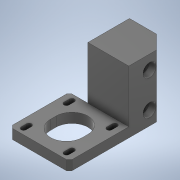
# Autodesk Inventor part: ymotorholder
Saved by Autodesk Inventor 2020.2 (Build 242310000, 310)
## iProperties
Created: 2020-08-06
Part Number: ymotorholder
Material: Generic
Document SubType Name: Modeling
Designer: JK
Density: 1 g/cm^3
Appearance: Smooth - Black
Author: JK
Autodesk Inventor part; units mm, degrees
ref_plane "YZ Plane" through (0, 0, 0) normal (1, 0, 0) x (0, 1, 0)
ref_plane "XZ Plane" through (0, 0, 0) normal (0, 1, 0) x (-1, 0, 0)
ref_plane "XY Plane" through (0, 0, 0) normal (0, 0, 1) x (1, 0, 0)
sketch "Sketch1" plane through (0, 0, 0) normal (0, 1, 0) x (-1, 0, 0)
  line L0 (-21.5, 21.5) -> (21.5, 21.5)
  line L1 (21.5, 21.5) -> (21.5, -21.5)
  line L2 (21.5, -21.5) -> (-21.5, -21.5)
  line L3 (-21.5, -21.5) -> (-21.5, 21.5)
  line L4 (-21.5, 21.5) -> (21.5, -21.5) construction
  line L5 (21.5, 21.5) -> (-21.5, -21.5) construction
  circle A0 centre (0, 0) radius 11.5
  circle A1 centre (15.5, 15.5) radius 1.8
  circle A2 centre (-15.5, 15.5) radius 1.8
  circle A3 centre (-15.5, -15.5) radius 1.8
  circle A4 centre (15.5, -15.5) radius 1.8
  dimension "d0" = 23
  dimension "d1" = 43
  dimension "d2" = 43
  dimension "d3" = 3.6
  dimension "d5" = 31
  dimension "d6" = 31
  constraints: 12 end point, 5 centre point, 4 point on line, 3 equal radius, 2 midpoint, 2 parallel, 2 vertical alignment, 1 coincident, 1 horizontal, 1 perpendicular
  measures "d0" diameter of A0
  measures "d1" distance of L1.end L2.end
  measures "d2" distance of L0.end L1.end
  measures "d3" diameter of A1
  measures "d5" distance of A4.centre A1.centre
  measures "d6" distance of A3.centre A4.centre
extrude "Extrusion1" add sketch "Sketch1" along normal blind 7
sketch "Sketch6" plane through (0, 0, 0) normal (0, -1, 0) x (1, 0, 0)
  line L0 (21.5, -21.5) -> (-21.5, -21.5) projected
  line L1 (-8, -21.5) -> (-8, -51.5)
  line L2 (21.5, -21.5) -> (-8, -21.5)
  line L3 (-8, -21.5) -> (-8, -51.5)
  line L4 (-8, -51.5) -> (21.5, -51.5)
  line L5 (21.5, -51.5) -> (21.5, -21.5)
  point P0 (0, 0)
  dimension "d26" = 8
  dimension "d27" = 30
  constraints: 10 end point, 2 parallel, 1 horizontal, 1 perpendicular, 1 point on line, 1 vertical
  measures "d26" distance from line of point (0, 0) L1
  measures "d27" distance of L1.start L1.end
extrude "Extrusion5" add sketch "Sketch6" against normal blind 45
chamfer "Chamfer1" distance 2 angle 45 3 edges at (21.5, 3.5, 21.5) (-21.5, 3.5, 21.5) (-21.5, 3.5, -21.5)
sketch "Sketch7" plane through (21.5, 0, -51.5) normal (1, 0, 0) x (0, 0, -1)
  circle A0 centre (-15, 35) radius 2.8
  circle A1 centre (-15, 10) radius 2.8
  line L0 (0, 0) -> (0, 45) projected
  line L1 (-71, 7) -> (-30, 7) projected
  line L2 (-71, 0) -> (0, 0) projected
  line L3 (-30, 45) -> (0, 45) projected
  point P0 (-51.5, 0)
  dimension "d33" = 5.6
  dimension "d34" = 5.6
  dimension "d35" = 15
  dimension "d37" = 10
  dimension "d38" = 10
  constraints: 2 centre point
  measures "d33" diameter of A0
  measures "d34" diameter of A1
  measures "d35" distance from line of L0 A0.centre
  measures "d37" distance from line of L2 A1.centre
  measures "d38" distance from line of L3 A0.centre
extrude "Extrusion6" cut sketch "Sketch7" against normal through all
sketch "Sketch8" plane through (21.5, 0, -51.5) normal (1, 0, 0) x (0, 0, -1)
  circle A0 centre (-15, 35) radius 2.8 projected
  circle A1 centre (-15, 35) radius 4.75
  circle A2 centre (-15, 10) radius 2.8 projected
  circle A3 centre (-15, 10) radius 4.75
  point P0 (-51.5, 0)
  dimension "d41" = 9.5
  dimension "d42" = 9.5
  constraints: 2 centre point, 2 coincident
  measures "d41" diameter of A1
  measures "d42" diameter of A3
extrude "Extrusion7" cut sketch "Sketch8" against normal blind 5 contours A0 | A1 | A2 | A3
chamfer "Chamfer2" distance 10 angle 45 1 edges at (21.5, 22.5, -51.5)
sketch "Sketch9" plane through (0, 0, 0) normal (0, -1, 0) x (1, 0, 0)
  line L0 (13.7, 17.5) -> (17.3, 17.5)
  line L1 (17.3, 17.5) -> (17.3, 13.5)
  line L2 (17.3, 13.5) -> (13.7, 13.5)
  line L3 (13.7, 13.5) -> (13.7, 17.5)
  circle A0 centre (15.5, 15.5) radius 1.8 projected
  line L4 (13.7, 17.5) -> (17.3, 13.5) construction
  line L5 (17.3, 17.5) -> (13.7, 13.5) construction
  line L6 (13.7, -13.5) -> (17.3, -13.5)
  line L7 (17.3, -13.5) -> (17.3, -17.5)
  line L8 (17.3, -17.5) -> (13.7, -17.5)
  line L9 (13.7, -17.5) -> (13.7, -13.5)
  circle A1 centre (15.5, -15.5) radius 1.8 projected
  line L10 (13.7, -13.5) -> (17.3, -17.5) construction
  line L11 (17.3, -13.5) -> (13.7, -17.5) construction
  line L12 (-17.3, 17.5) -> (-13.7, 17.5)
  line L13 (-13.7, 17.5) -> (-13.7, 13.5)
  line L14 (-13.7, 13.5) -> (-17.3, 13.5)
  line L15 (-17.3, 13.5) -> (-17.3, 17.5)
  circle A2 centre (-15.5, 15.5) radius 1.8 projected
  line L16 (-17.3, 17.5) -> (-13.7, 13.5) construction
  line L17 (-13.7, 17.5) -> (-17.3, 13.5) construction
  line L18 (-17.3, -13.5) -> (-13.7, -13.5)
  line L19 (-13.7, -13.5) -> (-13.7, -17.5)
  line L20 (-13.7, -17.5) -> (-17.3, -17.5)
  line L21 (-17.3, -17.5) -> (-17.3, -13.5)
  circle A3 centre (-15.5, -15.5) radius 1.8 projected
  line L22 (-17.3, -13.5) -> (-13.7, -17.5) construction
  line L23 (-13.7, -13.5) -> (-17.3, -17.5) construction
  circle A4 centre (15.5, 17.5) radius 1.8
  circle A5 centre (15.5, -17.5) radius 1.8
  circle A6 centre (15.5, -13.5) radius 1.8
  circle A7 centre (-15.5, -17.5) radius 1.8
  circle A8 centre (-15.5, -13.5) radius 1.8
  circle A9 centre (-15.5, 13.5) radius 1.8
  circle A10 centre (-15.5, 17.5) radius 1.8
  circle A11 centre (15.5, 13.5) radius 1.8
  point P0 (0, 0)
  point P1 (-17.3, 17.5)
  point P2 (13.7, 17.5)
  point P3 (17.3, 13.5)
  dimension "d48" = 4
  dimension "d49" = 4
  constraints: 48 end point, 16 midpoint, 8 parallel, 4 horizontal, 4 perpendicular, 3 point on line, 3 tangent, 2 horizontal alignment, 1 centre point, 21 other
  measures "d48" distance of L2.end L0.start
  measures "d49" distance of L6.end L7.end
extrude "Extrusion8" cut sketch "Sketch9" against normal blind 10
sketch "Sketch10" plane through (0, 0, 0) normal (0, -1, 0) x (1, 0, 0)
  line L0 (-11.5, 2) -> (11.5, 2)
  line L1 (11.5, 2) -> (11.5, -2)
  line L2 (11.5, -2) -> (-11.5, -2)
  line L3 (-11.5, -2) -> (-11.5, 2)
  line L4 (-11.5, 2) -> (11.5, -2) construction
  line L5 (11.5, 2) -> (-11.5, -2) construction
  circle A0 centre (0, -2) radius 11.5
  circle A1 centre (0, 2) radius 11.5
  circle A2 centre (0, 0) radius 11.5 projected
  point P0 (11.3248, 2)
  point P1 (-11.3248, 2)
  point P2 (-11.3248, -2)
  point P3 (11.3248, -2)
  point P4 (-11.5, 0)
  point P5 (11.5, 0)
  dimension "d52" = 4
  constraints: 12 end point, 4 midpoint, 2 parallel, 1 horizontal, 1 perpendicular, 1 tangent, 6 other
  measures "d52" distance of point (0, -2) point (0, 2)
extrude "Extrusion9" cut sketch "Sketch10" against normal blind 10
sketch "Sketch4" plane through (21.5, 0, 21.5) normal (1, 0, 0) x (0, 0, -1)
  line L0 (43, 45) -> (73, 45)
  line L1 (73, 45) -> (73, 0)
  line L2 (73, 0) -> (43, 0)
  line L3 (43, 0) -> (43, 45)
  line L4 (0, 0) -> (43, 0) projected
  line L5 (43, 0) -> (43, 7) projected
  point P0 (21.5, 0)
  dimension "d17" = 30
  dimension "d18" = 45
  constraints: 8 end point, 2 collinear, 2 parallel, 1 horizontal, 1 perpendicular
  measures "d17" distance between parallel lines of L1 L3
  measures "d18" distance of L0.end L1.end
sketch "Sketch5" plane through (21.5, 0, 21.5) normal (1, 0, 0) x (0, 0, -1)
  circle A0 centre (58, 33) radius 2.75
  circle A1 centre (58, 12) radius 2.75
  line L0 (73, 45) -> (43, 45) projected
  line L1 (0, 0) -> (73, 0) projected
  point P0 (21.5, 0)
  dimension "d21" = 12
  dimension "d22" = 12
  dimension "d23" = 5.5
  constraints: 2 centre point, 1 equal radius
  measures "d21" distance from line of L0 A0.centre
  measures "d22" distance from line of L1 A1.centre
  measures "d23" diameter of A0
body "Solid1"
